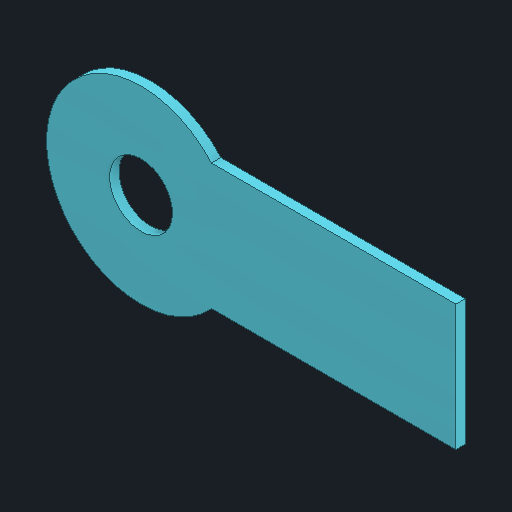
# Autodesk Inventor part: coxa_support_steel
Saved by Autodesk Inventor 2026 (Build 300175000, 175)
## iProperties
Created: 2026-04-25
Part Number: coxa_support_steel
Material: Сталь
Document SubType Name: Modeling
Designer: user
Mass: 202.749 g
Surface Area: 189.071 cm^2
Volume: 25.8279 cm^3
Density: 7.85 g/cm^3
Appearance: Серо-синий
Author: user
Autodesk Inventor part; units mm, degrees
ref_plane "YZ Plane" through (0, 0, 0) normal (1, 0, 0) x (0, 1, 0)
ref_plane "XZ Plane" through (0, 0, 0) normal (0, 1, 0) x (-1, 0, 0)
ref_plane "XY Plane" through (0, 0, 0) normal (0, 0, 1) x (1, 0, 0)
sketch "Эскиз3" plane through (0, 0, 0) normal (0, 0, 1) x (1, 0, 0)
  circle A0 centre (0, 0) radius 10
  arc A1 (22.3607, 20) -> (22.3607, -20) centre (0, 0) ccw
  line L0 (22.3607, 20) -> (100, 20)
  line L1 (100, 20) -> (100, -20)
  line L2 (100, -20) -> (22.3607, -20)
  line L3 (22.3607, -20) -> (22.3607, 20)
  dimension "d8" = 20
  dimension "d9" = 60
  dimension "d10" = 100
  dimension "d11" = 40
  constraints: 8 end point, 2 centre point, 2 coincident, 2 parallel, 2 point on circle, 1 horizontal, 1 perpendicular
  measures "d8" diameter of A0
  measures "d9" diameter of A1
  measures "d10" distance from line of point (0, 0) L1
  measures "d11" distance of L0.end L1.end
extrude "Выдавливание3" add sketch "Эскиз3" along normal blind 3
equation "\"d8\" = d_main_shaft"
equation "\"d10\" = length_coxa"
equation "\"d11\" = hight_coxa"
equation "\"d6\" = thickness_steel"
equation "\"tolerance_plazma\" = 0.1"
equation "\"thickness_steel\" = 3"
equation "\"d_main_screw_holes\" = 6.1"
equation "\"d_main_shaft\" = 20"
equation "\"thickness_profile_tibea\" = 3"
equation "\"hight_shaft_shift\" = 37"
equation "\"thickness_profile_femur\" = 3"
equation "\"width_shaft_shift\" = 35"
equation "\"width_flattened_surface\" = 12"
equation "\"length_coxa\" = 100"
equation "\"hight_coxa\" = 40"
